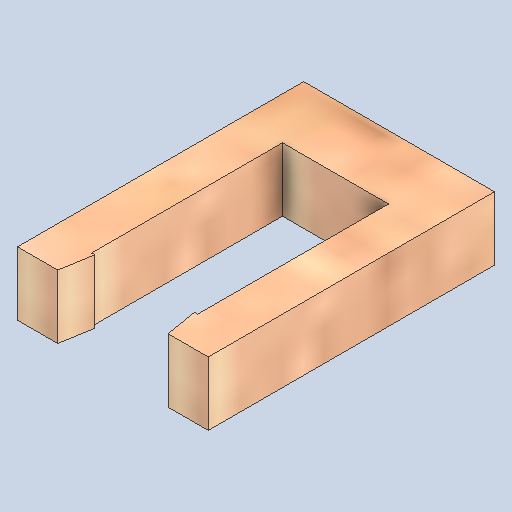
# Autodesk Inventor part: 夾持器
Saved by Autodesk Inventor 2024 (Build 280153000, 153)
## iProperties
Created: 2024-03-30
Part Number: 夾持器
Material: 木材 (樺木)
Document SubType Name: Modeling
Designer: USER
Density: 0.55 g/cm^3
Appearance: 樺木 - 天然拋光
Author: USER
Autodesk Inventor part; units mm, degrees
ref_plane "YZ Plane" through (0, 0, 0) normal (1, 0, 0) x (0, 1, 0)
ref_plane "XZ Plane" through (0, 0, 0) normal (0, 1, 0) x (-1, 0, 0)
ref_plane "XY Plane" through (0, 0, 0) normal (0, 0, 1) x (1, 0, 0)
sketch "草圖1" plane through (0, 0, 0) normal (0, 1, 0) x (-1, 0, 0)
  line L0 (0, 0) -> (9, 0)
  line L1 (9, 0) -> (9, 13.5)
  line L2 (0, 13.5) -> (0, 0)
  line L3 (2, 12) -> (2, 3)
  line L4 (2, 3) -> (7, 3)
  line L5 (7, 3) -> (7, 12)
  line L6 (9, 13.5) -> (7.1, 13.5)
  line L7 (7, 12) -> (6.85, 12)
  line L8 (7.1, 13.5) -> (6.85, 12)
  line L9 (4.5, 3) -> (4.5, 0)
  line L10 (0, 13.5) -> (1.9, 13.5)
  line L11 (2, 12) -> (2.15, 12)
  line L12 (1.9, 13.5) -> (2.15, 12)
  dimension "d0" = 13.5
  dimension "d1" = 9
  dimension "d2" = 5
  dimension "d3" = 9
  dimension "d4" = 1.5
  dimension "d5" = 2
  dimension "d6" = 1.9
  dimension "d7" = 0.15
  dimension "d8" = 2
  dimension "d9" = 5
  constraints: 26 end point, 4 parallel, 3 horizontal, 2 midpoint, 2 symmetric about line, 1 perpendicular
  measures "d0" distance of L2.start L0.start
  measures "d1" distance of L0.start L0.end
  measures "d2" distance of L3.end L4.end
  measures "d3" distance of L3.start L3.end
  measures "d4" vertical distance of L1.end L5.end
  measures "d5" horizontal distance of L1.end L5.end
  measures "d6" distance of L1.end L6.end
  measures "d7" distance of L5.end L7.end
  measures "d8" distance from line of L2 L3.end
  measures "d9" distance between parallel lines of L5 L3
extrude "擠出1" add sketch "草圖1" along normal blind 3
